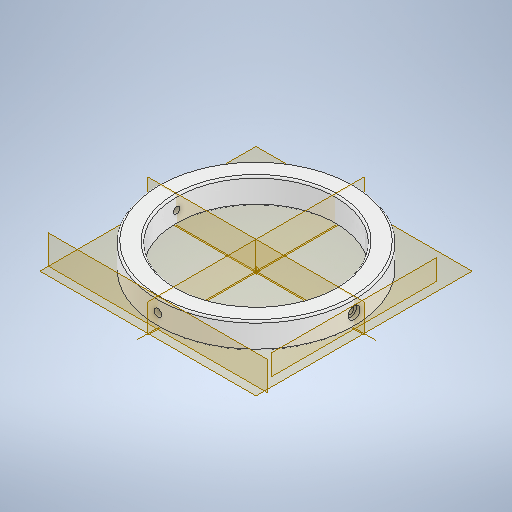
# Autodesk Inventor part: o-ring
Saved by Autodesk Inventor 2025.2 (Build 292293000, 293)
## iProperties
Created: 2025-03-14
Part Number: o-ring
Material: ABS Plastic
Document SubType Name: Modeling
Designer: yehorderehus
Density: 1.06 g/cm^3
Appearance: Smooth - White
Mass: 43.4821 g
Surface Area: 141.424 cm^2
Volume: 41.0208 cm^3
Author: yehorderehus
Autodesk Inventor part; units mm, degrees
note: some values were not read from the file. Chosen so that the rebuilt part matches the saved one: direction of "Hole1".
sketch "Sketch1" plane through (0, 0, 0) normal (0, 1, 0) x (-1, 0, 0)
  circle A0 centre (0, 0) radius 42.4
  circle A1 centre (0, 0) radius 52.4
  dimension "d0" = 84.8
  dimension "d1" = 10
  constraints: 2 centre point, 2 coincident
  measures "d0" diameter of A0
  measures "d1" radial gap between concentric circles of A0 A1
extrude "Extrusion1" add sketch "Sketch1" along normal blind 14
fillet "Fillet1" radius 1 4 edges at (52.4, 14, 0) (42.4, 14, 0) (52.4, 0, 0) (42.4, 0, 0)
ref_plane "Work Plane1" through (52.4, 0, 0) normal (1, 0, 0) x (0, 1, 0)
sketch "Sketch2" plane through (52.4, 0, 0) normal (1, 0, 0) x (0, 1, 0)
  line L0 (0, 73.36) -> (0, -73.36) projected
  point P0 (0, 0)
  point P1 (7, 0)
  dimension "d5" = 7
  measures "d5" distance from line of L0 point (7, 0)
hole "Hole1" at (52.4, 7, 0) direction (-1, 0, 0) diameter 3.4 end up to surface counterbore diameter 6.4 counterbore depth 2
pattern_circular "Circular Pattern1" count 2 over 360 about axis through (0, -10, 0) along (0, 1, 0) of "Hole1"
ref_plane "Work Plane7" through (0, 0, 52.4) normal (0, 0, 1) x (1, 0, 0)
sketch "Sketch8" plane through (0, 0, 52.4) normal (0, 0, 1) x (1, 0, 0)
  line L0 (-73.36, 0) -> (73.36, 0) projected
  point P0 (0, 0)
  point P1 (0, 7)
  dimension "d53" = 7
  measures "d53" distance from line of L0 point (0, 7)
hole "Hole5" at (0, 7, 52.4) direction (0, 0, -1) diameter 4 depth 5.8
pattern_circular "Circular Pattern4" count 2 over 360 about axis through (0, -10, 0) along (0, 1, 0) of "Hole5"
equation "\"d5\" = 0.5 * d2"
equation "\"d53\" = 0.5 * d2"
equation "\"d2\" = 14"
body "Solid1"
